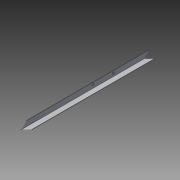
# Autodesk Inventor part: Shooter Middle Support Bar
Saved by Autodesk Inventor 2014 SP1 (Build 180222100, 222)
## iProperties
Created: 2013-12-13
Part Number: Shooter Middle Support Bar
Material: Aluminum 6061
Document SubType Name: Modeling
Designer: Moses
Mass: 31.7744 g
Surface Area: 304.244 cm^2
Volume: 11.7249 cm^3
Density: 2.71 g/cm^3
Appearance: Aluminum - Flat
Author: Moses
Autodesk Inventor part; units mm, degrees
ref_plane "YZ Plane" through (0, 0, 0) normal (1, 0, 0) x (0, 1, 0)
ref_plane "XZ Plane" through (0, 0, 0) normal (0, 1, 0) x (-1, 0, 0)
ref_plane "XY Plane" through (0, 0, 0) normal (0, 0, 1) x (1, 0, 0)
sketch "Sketch1" plane through (0, 0, 0) normal (0, 0, 1) x (1, 0, 0)
  line L0 (0, 0) -> (0, 15.875)
  line L1 (0, 15.875) -> (0.7937, 15.875)
  line L2 (0.7937, 15.875) -> (0.7938, 0.7937)
  line L3 (0.7938, 0.7937) -> (15.875, 0.7937)
  line L4 (15.875, 0.7937) -> (15.875, 0)
  line L5 (15.875, 0) -> (0, 0)
  dimension "d0" = 15.875
  dimension "d1" = 0.7937
  constraints: 12 end point, 3 horizontal, 3 vertical, 2 perpendicular
  measures "d0" distance of L0.start L0.end
  measures "d1" distance of L0.end L1.end
extrude "Extrusion1" add sketch "Sketch1" along normal blind 481.8063
sketch "Sketch2" plane through (0, 0, 0) normal (-1, 0, 0) x (0, 0, 1)
  circle A0 centre (46.4113, 9.6145) radius 3.3782 projected
  circle A1 centre (158.9314, 9.6145) radius 3.3782 projected
  circle A2 centre (701.675, 21.658) radius 3.3782 construction
  circle A3 centre (701.675, 43.7923) radius 3.3782 construction
  circle A4 centre (701.675, 32.7252) radius 3.3782 construction
  circle A5 centre (701.675, 10.5909) radius 3.3782 projected
  line L0 (366.395, 51.5938) -> (366.395, 0.7938) construction
  line L1 (708.025, 0.7938) -> (366.395, 0.7938) construction
  line L2 (708.025, 51.5938) -> (708.025, 0.7938) construction
  line L3 (366.395, 51.5938) -> (708.025, 51.5938) construction
  circle A6 centre (219.075, 21.658) radius 3.3782 construction
  circle A7 centre (219.075, 43.7923) radius 3.3782 construction
  circle A8 centre (219.075, 32.7252) radius 3.3782 construction
  circle A9 centre (219.075, 10.5909) radius 3.3782 projected
  line L4 (262.255, 51.5938) -> (262.255, 0.7938) construction
  line L5 (212.725, 0.7938) -> (262.255, 0.7938) construction
  line L6 (212.725, 0.7938) -> (212.725, 51.5938) construction
  line L7 (212.725, 51.5938) -> (262.255, 51.5938) construction
  line L8 (0, 0) -> (0, 15.875) projected
  line L9 (481.8063, 15.875) -> (481.8063, 0) projected
  line L10 (19.05, -173.8312) -> (19.05, -103.9812) construction
  line L11 (19.05, -103.9812) -> (285.75, -103.9812) construction
  line L12 (285.75, -103.9812) -> (285.75, -173.8312) construction
  line L13 (285.75, -173.8312) -> (19.05, -173.8312) construction
  line L14 (38.1, -294.4812) -> (38.1, -265.9062) construction
  line L15 (38.1, -265.9062) -> (285.75, -265.9062) construction
  line L16 (285.75, -265.9062) -> (285.75, -294.4812) construction
  line L17 (285.75, -294.4812) -> (38.1, -294.4812) construction
  circle A10 centre (593.725, 76.9938) radius 3.3782 construction
  circle A11 centre (314.325, -202.4062) radius 3.3782 construction
  circle A12 centre (454.025, 76.9938) radius 3.3782 construction
  circle A13 centre (417.4958, -17.1968) radius 3.3782 construction
  circle A14 centre (408.5156, -26.1771) radius 3.3782 construction
  circle A15 centre (516.3297, -116.0307) radius 3.3782 construction
  circle A16 centre (507.3495, -125.011) radius 3.3782 construction
  circle A17 centre (259.0504, -62.7062) radius 3.3782 construction
  circle A18 centre (314.325, -62.7062) radius 3.3782 construction
  line L18 (191.2043, 15.9645) -> (11.4863, 15.9645) construction
  line L19 (11.4863, 15.9645) -> (11.4863, 0.7938) construction
  line L20 (11.4863, 0.7938) -> (0, 0.7938) construction
  line L21 (0, 0.7938) -> (0, -316.7062) construction
  line L22 (0, -316.7062) -> (307.975, -316.7062) construction
  line L23 (307.975, -316.7062) -> (307.975, -208.7562) construction
  line L24 (307.975, -208.7562) -> (314.325, -208.7562) construction
  arc A19 (314.325, -208.7562) -> (600.075, 76.9938) centre (314.325, 76.9938) ccw construction
  line L25 (600.075, 76.9938) -> (600.075, 83.3438) construction
  line L26 (600.075, 83.3438) -> (587.375, 83.3438) construction
  line L27 (587.375, 83.3438) -> (587.375, 76.9938) construction
  arc A20 (314.325, -196.0562) -> (587.375, 76.9938) centre (314.325, 76.9938) ccw construction
  line L28 (314.325, -196.0562) -> (314.325, -69.0562) construction
  arc A21 (314.325, -69.0562) -> (460.375, 76.9938) centre (314.325, 76.9938) ccw construction
  line L29 (460.375, 76.9938) -> (460.375, 83.3438) construction
  line L30 (460.375, 83.3438) -> (447.675, 83.3438) construction
  line L31 (447.675, 83.3438) -> (447.675, 76.9938) construction
  arc A22 (314.325, -56.3562) -> (447.675, 76.9938) centre (314.325, 76.9938) ccw construction
  line L32 (314.325, -56.3562) -> (193.675, 0.7938) construction
  line L33 (193.675, 0.7938) -> (193.675, 13.4938) construction
  line L34 (193.675, 13.4938) -> (191.2043, 15.9645) construction
  line L35 (19.05, -215.1062) -> (19.05, -186.5312) construction
  line L36 (19.05, -186.5312) -> (285.75, -186.5312) construction
  line L37 (285.75, -186.5312) -> (285.75, -215.1062) construction
  line L38 (285.75, -215.1062) -> (19.05, -215.1062) construction
  line L39 (25.4, -253.2062) -> (25.4, -281.7812) construction
  line L40 (25.4, -281.7812) -> (19.05, -281.7812) construction
  line L41 (19.05, -281.7812) -> (19.05, -253.2062) construction
  line L42 (19.05, -253.2062) -> (12.7, -253.2062) construction
  line L43 (12.7, -253.2062) -> (12.7, -227.8062) construction
  line L44 (12.7, -227.8062) -> (215.9, -227.8062) construction
  line L45 (215.9, -227.8062) -> (215.9, -253.2062) construction
  line L46 (215.9, -253.2062) -> (25.4, -253.2062) construction
  line L47 (25.4, 6.4395) -> (25.4, -62.7062) construction
  line L48 (25.4, -62.7062) -> (215.9, -62.7062) construction
  line L49 (215.9, -62.7062) -> (215.9, -88.1062) construction
  line L50 (215.9, -88.1062) -> (12.7, -88.1062) construction
  line L51 (12.7, -88.1062) -> (12.7, -62.7062) construction
  line L52 (12.7, -62.7062) -> (19.05, -62.7062) construction
  line L53 (19.05, -62.7062) -> (19.05, 6.4395) construction
  line L54 (19.05, 6.4395) -> (25.4, 6.4395) construction
  circle A23 centre (238.125, -310.3562) radius 3.3782 construction
  circle A24 centre (219.075, -310.3562) radius 3.3782 construction
  circle A25 centre (46.4113, 9.6145) radius 3.3782 construction
  circle A26 centre (158.9314, 9.6145) radius 3.3782 construction
  arc A27 (314.325, -62.7062) -> (454.025, 76.9938) centre (314.325, 76.9938) ccw construction
  line L55 (481.8063, 7.9375) -> (0, 7.9375) construction
  circle A28 centre (435.7636, 7.9375) radius 3.3782
  dimension "d6" = 6.7564
  constraints: 4 point on circle, 2 centre point, 2 end point, 2 midpoint, 1 point on line
  measures "d6" diameter of A28
extrude "Extrusion2" cut sketch "Sketch2" against normal through all
body "Solid1"
